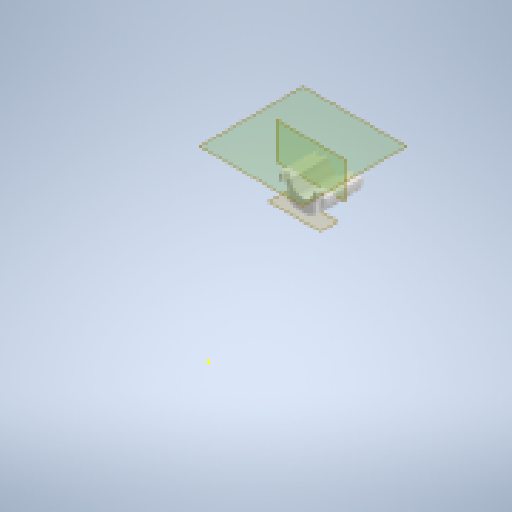
# Autodesk Inventor part: верх штуки для подшипников
Saved by Autodesk Inventor 2024.2 (Build 282272000, 272)
## iProperties
Created: 2025-11-24
Part Number: верх штуки для подшипников
Material: Типовые
Document SubType Name: Modeling
Designer: katya_notebook
Density: 1 g/cm^3
Appearance: По умолчанию
Author: katya_notebook
Autodesk Inventor part; units mm, degrees
ref_plane "YZ Plane" through (0, 0, 0) normal (1, 0, 0) x (0, 1, 0)
ref_plane "XZ Plane" through (0, 0, 0) normal (0, 1, 0) x (-1, 0, 0)
ref_plane "XY Plane" through (0, 0, 0) normal (0, 0, 1) x (1, 0, 0)
ref_plane "РабПлоскость1" through (-89.0227, 116.8233, -154.317) normal (0, 0, -1) x (-1, 0, 0)
sketch "Эскиз1" plane through (-89.0227, 116.8233, -154.317) normal (0, 0, -1) x (-1, 0, 0)
  arc A0 (7.1, -10.5) -> (-7.1, -10.5) centre (0, -10.5) ccw projected
  line L0 (7.1, -10.5) -> (15, -10.5) projected
  line L1 (15, -10.5) -> (15, 7.5) projected
  line L2 (15, 7.5) -> (17, 7.5) projected
  line L3 (20, 10.5) -> (-20, 10.5) projected
  line L4 (-17, 7.5) -> (-15, 7.5) projected
  line L5 (-15, 7.5) -> (-15, -10.5) projected
  line L6 (-15, -10.5) -> (-7.1, -10.5) projected
  circle A1 centre (0, -10.5) radius 15
  line L7 (15, -10.5) -> (-15, -10.5)
  circle A2 centre (0, -10.5) radius 7 projected
  circle A3 centre (0, -10.5) radius 7.1
  line L8 (15, -10.5) -> (-15, -10.5)
  line L9 (20, 10.5) -> (17, 7.5) projected
  line L10 (-17, 7.5) -> (-20, 10.5) projected
  point P0 (-89.0227, -116.8233)
  point P1 (-7.1, -10.5)
  constraints: 4 end point, 2 coincident, 2 point on circle, 1 centre point, 1 horizontal, 3 other
extrude "Выдавливание1" add sketch "Эскиз1" against normal blind 5.8 contours L0 A1 L6 A3
ref_plane "РабПлоскость2" through (-89.2672, 127.3233, -149.317) normal (0, -1, 0) x (1, 0, 0)
ref_plane "РабПлоскость3" through (-89.0227, 91.3233, -154.317) normal (0, 1, 0) x (1, 0, 0)
sketch "Эскиз3" plane through (-89.2672, 127.3233, -149.317) normal (0, -1, 0) x (1, 0, 0)
  point P0 (89.2672, 149.317)
sketch "Эскиз4" plane through (-89.0227, 91.3233, -154.317) normal (0, 1, 0) x (1, 0, 0)
  circle A0 centre (-11.518, -0.8) radius 2.025
  circle A1 centre (10.9976, -0.8) radius 2.025
  circle A2 centre (10.9976, -0.8) radius 3.25
  line L0 (8.1777, 0.8159) -> (10.987, 2.45)
  line L1 (10.987, 2.45) -> (13.8069, 0.8341)
  line L2 (13.8069, 0.8341) -> (13.8174, -2.4159)
  line L3 (13.8174, -2.4159) -> (11.0081, -4.05)
  line L4 (11.0081, -4.05) -> (8.1883, -2.4341)
  line L5 (8.1883, -2.4341) -> (8.1777, 0.8159)
  circle A3 centre (-11.518, -0.8) radius 3.25
  line L6 (-14.3346, 0.8215) -> (-11.5221, 2.45)
  line L7 (-11.5221, 2.45) -> (-8.7055, 0.8285)
  line L8 (-8.7055, 0.8285) -> (-8.7014, -2.4215)
  line L9 (-8.7014, -2.4215) -> (-11.514, -4.05)
  line L10 (-11.514, -4.05) -> (-14.3306, -2.4285)
  line L11 (-14.3306, -2.4285) -> (-14.3346, 0.8215)
  point P0 (89.0227, -154.317)
  point P1 (-9.5168, -5)
  point P2 (-13.3499, -5.8)
  dimension "d19" = 6.5
  constraints: 24 end point, 4 coincident, 2 centre point, 36 other
sketch "Эскиз5" plane through (-89.0227, 116.8233, -154.317) normal (0, 0, -1) x (-1, 0, 0)
  arc A0 (-15, -10.5) -> (15, -10.5) centre (0, -10.5) ccw projected
  arc A1 (-7.1, -10.5) -> (7.1, -10.5) centre (0, -10.5) ccw projected
  line L0 (-7.1, -10.5) -> (-15, -10.5) projected
  line L1 (15, -10.5) -> (7.1, -10.5) projected
  point P0 (-89.0227, -116.8233)
ref_plane "РабПлоскость4" through (-119.2672, 76.6183, -172.817) normal (0, 0, 1) x (1, 0, 0)
extrude "Выдавливание5" add sketch "Эскиз5" along normal up to surface (18.5 mm away)
sketch "Эскиз6" plane through (-81.9227, 106.3233, -148.517) normal (0, 1, 0) x (1, 0, 0)
  spline S0 degree 3 poles (3.9004, 2.9999) (3.7245, 2.9999) (3.4489, 3.0214) (2.9324, 3.2367) (2.7005, 3.3696) (2.2383, 3.836) (2.1143, 4.0825) (1.9216, 4.5561) (1.8983, 4.8272) (1.9018, 5.2007) (1.9271, 5.4608) (2.115, 5.9172) (2.2283, 6.1414) (2.6589, 6.5988) (2.8813, 6.7317) (3.3428, 6.9462) (3.5921, 6.9833) (3.938, 7.0077) (4.1964, 7.0052) (4.7621, 6.8239) (4.993, 6.6978) (5.3793, 6.3686) (5.5529, 6.1613) (5.836, 5.6049) (5.8802, 5.3338) (5.9139, 4.8965) (5.8839, 4.6393) (5.7537, 4.2295) (5.6627, 4.0097) (5.3189, 3.5657) (5.1225, 3.3931) (4.7049, 3.1558) (4.5337, 3.0993) (4.2495, 3.0231) (4.0752, 3) (3.9004, 2.9999) knots 0 0 0 0 0.05278 0.05278 0.086326 0.086326 0.123204 0.123204 0.191125 0.191125 0.256265 0.256265 0.291032 0.291032 0.325738 0.325738 0.381328 0.381328 0.440927 0.440927 0.488647 0.488647 0.532429 0.532429 0.584012 0.584012 0.657631 0.657631 0.707027 0.707027 0.750679 0.750679 0.786548 0.786548 0.838987 0.838987 0.838987 0.838987 projected
  line L0 (7.9, 0) -> (7.9, 10) projected
  line L1 (7.9, 28.5) -> (7.9, 10) projected
  spline S1 degree 3 poles (-18.6169, 3) (-18.8661, 3) (-19.1174, 3.0465) (-19.5436, 3.2165) (-19.7767, 3.3398) (-20.1687, 3.7191) (-20.3359, 3.938) (-20.5737, 4.4851) (-20.6126, 4.7587) (-20.621, 5.202) (-20.5814, 5.4471) (-20.4, 5.9515) (-20.2582, 6.1524) (-19.9577, 6.5137) (-19.7534, 6.6562) (-19.3614, 6.8745) (-19.1056, 6.9583) (-18.5778, 7.0163) (-18.3108, 6.9948) (-17.7812, 6.8389) (-17.5504, 6.709) (-17.1606, 6.3952) (-16.9882, 6.1918) (-16.7635, 5.7779) (-16.6604, 5.5273) (-16.5953, 4.8865) (-16.6419, 4.6209) (-16.754, 4.2513) (-16.8422, 4.0327) (-17.1223, 3.6603) (-17.294, 3.4644) (-17.7748, 3.1712) (-17.9576, 3.1063) (-18.2654, 3.0232) (-18.4408, 3) (-18.6169, 3) knots 0 0 0 0 0.074777 0.074777 0.132907 0.132907 0.176214 0.176214 0.221242 0.221242 0.273328 0.273328 0.334855 0.334855 0.445019 0.445019 0.599494 0.599494 0.747069 0.747069 0.901689 0.901689 1.065475 1.065475 1.190217 1.190217 1.309721 1.309721 1.411319 1.411319 1.472242 1.472242 1.514996 1.514996 1.5678 1.5678 1.5678 1.5678 projected
  spline S2 degree 3 poles (1.8953, 19.3009) (1.8944, 19.3863) (1.8996, 19.5644) (2.0298, 20.0176) (2.1169, 20.2293) (2.4403, 20.7217) (2.6648, 20.8786) (2.9132, 21.0563) (3.1329, 21.1685) (3.5962, 21.2734) (3.8627, 21.3137) (4.1292, 21.2939) (4.4485, 21.2503) (5.0812, 20.9371) (5.2298, 20.8085) (5.5261, 20.5131) (5.6407, 20.3138) (5.8212, 19.8892) (5.8776, 19.6525) (5.9089, 19.3478) (5.9108, 19.063) (5.6799, 18.3006) (5.5185, 18.1178) (5.3603, 17.9264) (5.2248, 17.7844) (4.7267, 17.4265) (4.3507, 17.3562) (3.9904, 17.2726) (3.8261, 17.2836) (3.4517, 17.3475) (3.1747, 17.4305) (2.784, 17.6252) (2.5802, 17.7693) (2.1778, 18.2343) (2.0816, 18.439) (1.9561, 18.8227) (1.8978, 19.0803) (1.8953, 19.3009) knots -0.617581 -0.617581 -0.617581 -0.617581 -0.591947 -0.591947 -0.573073 -0.573073 -0.540222 -0.540222 -0.491682 -0.491682 -0.466072 -0.466072 -0.460987 -0.460987 -0.456841 -0.456841 -0.449459 -0.449459 -0.440712 -0.440712 -0.435051 -0.435051 -0.427631 -0.427631 -0.418066 -0.418066 -0.393854 -0.393854 -0.318016 -0.318016 -0.225773 -0.225773 -0.149383 -0.149383 -0.066183 -0.066183 0 0 0 0
  spline S3 degree 3 poles (-20.1358, 20.5982) (-19.9784, 20.7756) (-19.7373, 20.9815) (-19.2566, 21.217) (-19.0243, 21.2678) (-18.5989, 21.3096) (-18.3448, 21.3092) (-17.7198, 21.1156) (-17.5007, 20.9708) (-17.0322, 20.5784) (-16.879, 20.2945) (-16.7767, 20.0958) (-16.6834, 19.8667) (-16.6099, 19.4343) (-16.5909, 19.1881) (-16.7143, 18.6599) (-16.8009, 18.3991) (-17.121, 17.9518) (-17.3048, 17.7698) (-17.7894, 17.4486) (-18.0589, 17.3712) (-18.5717, 17.273) (-18.8341, 17.303) (-19.1764, 17.3757) (-19.3925, 17.4419) (-19.6812, 17.5968) (-19.8978, 17.7223) (-20.2684, 18.178) (-20.4032, 18.3633) (-20.5197, 18.6522) (-20.6106, 18.8835) (-20.6111, 19.6503) (-20.535, 19.8971) (-20.3432, 20.3552) (-20.1819, 20.5462) (-20.1358, 20.5982) knots -1.840358 -1.840358 -1.840358 -1.840358 -1.769222 -1.769222 -1.709875 -1.709875 -1.656566 -1.656566 -1.604902 -1.604902 -1.500987 -1.500987 -1.176684 -1.176684 -0.960047 -0.960047 -0.825926 -0.825926 -0.728108 -0.728108 -0.603604 -0.603604 -0.389887 -0.389887 -0.189621 -0.189621 -0.087541 -0.087541 -0.045854 -0.045854 -0.032602 -0.032602 -0.020855 -0.020855 0 0 0 0
  point P0 (81.9227, -148.517)
  point P1 (3.9004, 2.9999)
  point P2 (7.9, 14.25)
  point P3 (-18.6169, 3)
  constraints: 1 point on line, 4 other
extrude "Выдавливание6" cut sketch "Эскиз6" against normal blind 21.25 contours S2 | S3
extrude "Выдавливание3" cut sketch "Эскиз4" along normal blind 10 contours A0 | A1 | L2 L3 L4 L5 L0 L1 | L8 L9 L10 L11 L6 L7
sketch "Эскиз7" plane through (-89.0227, 91.3233, -154.317) normal (0, 1, 0) x (1, 0, 0)
  line L0 (13.7865, -5.8) -> (13.7865, -3.3744) projected
  line L1 (13.7865, -3.3744) -> (10.9719, -1.7494) projected
  line L2 (10.9719, -1.7494) -> (8.1574, -3.3744) projected
  line L3 (8.1574, -3.3744) -> (8.1574, -5.8) projected
  line L4 (8.1574, -6.6244) -> (10.9719, -8.2494) projected
  line L5 (10.9719, -8.2494) -> (13.7865, -6.6244) projected
  line L6 (-14.1421, -3.2792) -> (-14.1421, -5.8) projected
  line L7 (-11.5035, -1.7558) -> (-14.1421, -3.2792) projected
  line L8 (-8.689, -3.3808) -> (-11.5035, -1.7558) projected
  line L9 (-8.689, -5.8) -> (-8.689, -3.3808) projected
  line L10 (-11.5035, -8.2558) -> (-8.689, -6.6308) projected
  line L11 (-14.1421, -6.7324) -> (-11.5035, -8.2558) projected
  line L12 (-15, -5.8) -> (-15, 18.5) projected
  line L13 (-15, 4.25) -> (5.6318, 4.25)
  line L14 (13.7865, 15.1244) -> (13.7865, 11.8744)
  line L15 (13.7865, 11.8744) -> (10.9719, 10.2494)
  line L16 (10.9719, 10.2494) -> (8.1574, 11.8744)
  line L17 (8.1574, 11.8744) -> (8.1574, 15.1244)
  line L18 (8.1574, 15.1244) -> (10.9719, 16.7494)
  line L19 (10.9719, 16.7494) -> (13.7865, 15.1244)
  line L20 (-14.1421, 11.7792) -> (-14.1421, 15.2324)
  line L21 (-11.5035, 10.2558) -> (-14.1421, 11.7792)
  line L22 (-8.689, 11.8808) -> (-11.5035, 10.2558)
  line L23 (-8.689, 15.1308) -> (-8.689, 11.8808)
  line L24 (-11.5035, 16.7558) -> (-8.689, 15.1308)
  line L25 (-14.1421, 15.2324) -> (-11.5035, 16.7558)
  point P0 (89.0227, -154.317)
  point P1 (-11.5169, 15.5)
  point P2 (11.0004, 15.5001)
  point P3 (-9.3627, -7.088)
  point P4 (-9.3627, 15.588)
  dimension "d16" = 14.25
  constraints: 26 end point, 13 symmetric about line, 1 horizontal, 1 point on line, 3 other
  measures "d16" distance of L12.end L13.start
extrude "Выдавливание7" cut sketch "Эскиз7" along normal up to surface (10 mm away)
sketch "Эскиз2" plane through (-89.2672, 127.3233, -149.317) normal (0, -1, 0) x (1, 0, 0)
  line L0 (-14.7555, -5) -> (15.2445, -5) projected
  line L1 (15.2445, -5) -> (15.2445, 0.8) projected
  line L2 (-6.8555, 0.8) -> (7.3445, 0.8) projected
  line L3 (-0.0139, 0.8) -> (-0.0139, -5)
  circle A0 centre (-11.2735, -4.2) radius 2.025
  circle A1 centre (11.2421, -4.2) radius 2.025
  point P0 (89.2672, 149.317)
  constraints: 2 centre point, 2 end point, 2 point on line, 1 perpendicular, 4 other
extrude "Выдавливание8" cut sketch "Эскиз2" along normal blind 51.5
